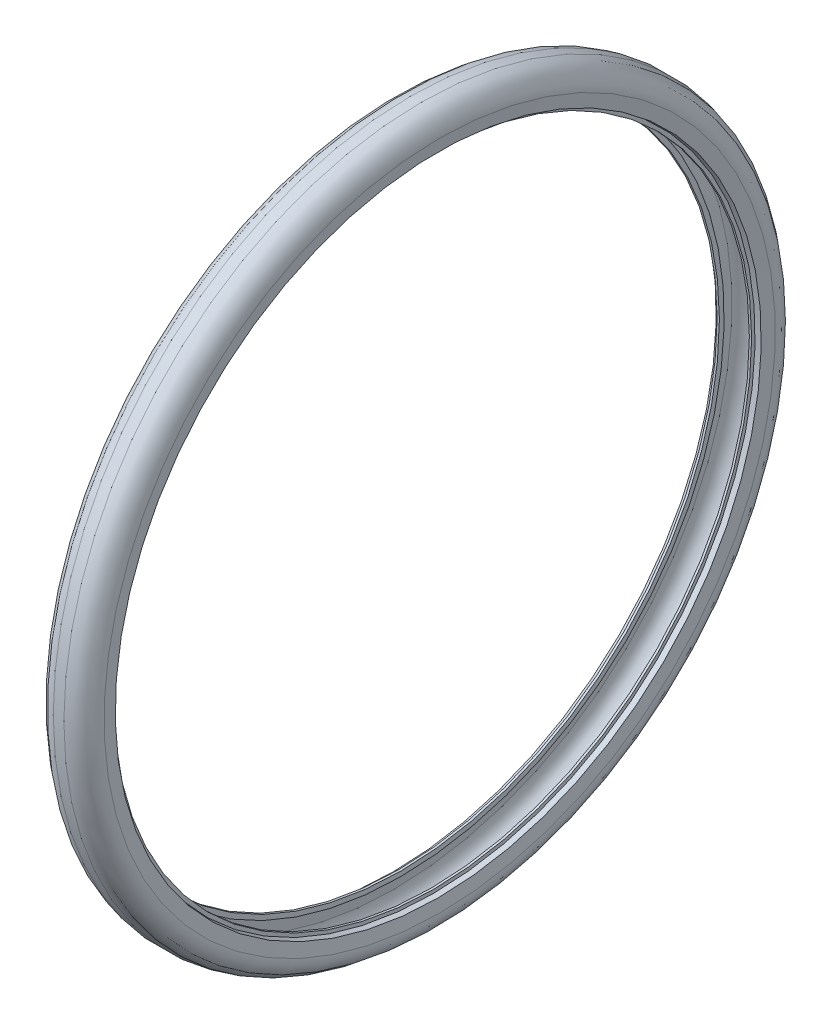
# Autodesk Inventor part: llanta_ruta_2
Saved by Autodesk Inventor 2021 (Build 250183000, 183)
## iProperties
Created: 2021-07-05
Part Number: llanta_ruta_2
Material: Generic
Document SubType Name: Modeling
Designer: j2seb
Density: 1 g/cm^3
Appearance: Default
Author: j2seb
Autodesk Inventor part; units mm, degrees
ref_plane "YZ Plane" through (0, 0, 0) normal (1, 0, 0) x (0, 1, 0)
ref_plane "XZ Plane" through (0, 0, 0) normal (0, 1, 0) x (-1, 0, 0)
ref_plane "XY Plane" through (0, 0, 0) normal (0, 0, 1) x (1, 0, 0)
sketch "Sketch1" plane through (0, 0, 0) normal (0, 0, 1) x (1, 0, 0)
  line L0 (19.6559, -282.1366) -> (20.8927, -293.0931)
  arc A0 (4.6301, -311.9883) -> (20.8927, -293.0931) centre (4, -295) ccw
  line L1 (4.6301, -311.9883) -> (0, -311.9883)
  line L2 (19.6559, -282.1366) -> (15.0778, -281.3613)
  line L3 (15.0778, -281.3613) -> (15.0778, -278.3008)
  line L4 (15.0778, -278.3008) -> (13.0778, -278.3008)
  line L5 (13.0778, -278.3008) -> (13.0778, -282.4918)
  line L6 (13.0778, -282.4918) -> (17.6747, -283.4364)
  line L7 (17.6747, -283.4364) -> (18.9881, -295.072)
  arc A1 (4, -309.9883) -> (18.9881, -295.072) centre (4, -295) ccw
  line L8 (4, -309.9883) -> (0, -309.9883)
  line L9 (0, -311.9883) -> (0, 0)
  line L10 (0, 0) -> (0, -311.9883) construction
  line L11 (-19.6559, -282.1366) -> (-20.8927, -293.0931)
  arc A2 (-20.8927, -293.0931) -> (-4.6301, -311.9883) centre (-4, -295) ccw
  line L12 (-4.6301, -311.9883) -> (0, -311.9883)
  line L13 (-19.6559, -282.1366) -> (-15.0778, -281.3613)
  line L14 (-15.0778, -281.3613) -> (-15.0778, -278.3008)
  line L15 (-15.0778, -278.3008) -> (-13.0778, -278.3008)
  line L16 (-13.0778, -278.3008) -> (-13.0778, -282.4918)
  line L17 (-13.0778, -282.4918) -> (-17.6747, -283.4364)
  line L18 (-17.6747, -283.4364) -> (-18.9881, -295.072)
  arc A3 (-18.9881, -295.072) -> (-4, -309.9883) centre (-4, -295) ccw
  line L19 (-4, -309.9883) -> (0, -309.9883)
  line L20 (-35.0226, 0) -> (35.0226, 0) projected
  dimension "d2" = 17
  dimension "d3" = 295
  dimension "d4" = 4
  dimension "d5" = 2
  dimension "d6" = 2
  dimension "d8" = 2
  constraints: 40 end point, 12 symmetric about line, 8 point on circle, 4 centre point, 3 vertical alignment, 2 parallel, 2 perpendicular, 2 tangent, 2 vertical, 1 collinear, 1 concentric, 1 horizontal, 2 other
  measures "d2" radius of A0
  measures "d3" vertical distance of L9.end A0.centre
  measures "d4" horizontal distance of L9.end A0.centre
  measures "d5" distance of L3.end L4.end
  measures "d6" angle of L6 L2
  measures "d8" distance between parallel lines of L1 L8
revolve "Revolution1" add sketch "Sketch1" angle 360 about axis through (-10, 0, 0) along (1, 0, 0)
body "Solid1"
